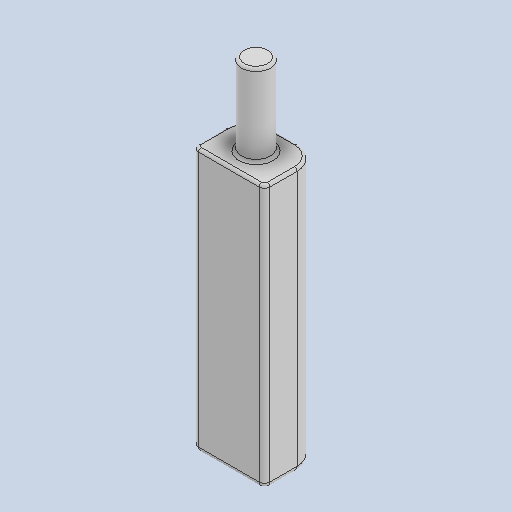
# Autodesk Inventor part: ArmLength
Saved by Autodesk Inventor 2025.2 (Build 292293000, 293)
## iProperties
Created: 2025-02-05
Part Number: ArmLength
Material: Generic
Document SubType Name: Modeling
Designer: andre
Density: 1 g/cm^3
Appearance: Default
Author: andre
Autodesk Inventor part; units mm, degrees
ref_plane "YZ Plane" through (0, 0, 0) normal (1, 0, 0) x (0, 1, 0)
ref_plane "XZ Plane" through (0, 0, 0) normal (0, 1, 0) x (-1, 0, 0)
ref_plane "XY Plane" through (0, 0, 0) normal (0, 0, 1) x (1, 0, 0)
sketch "Sketch1" plane through (0, 0, 0) normal (0, 0, 1) x (1, 0, 0)
  arc A0 (6.6, 0) -> (-2.5948, -6.0685) centre (0, 0) ccw construction
  circle A1 centre (0, 0) radius 6.6
  line L0 (-6.5674, -56.9808) -> (6.5674, -56.9808)
  line L1 (6.5674, -56.9808) -> (6.5674, 56.9808)
  line L2 (6.5674, 56.9808) -> (-6.5674, 56.9808)
  line L3 (-6.5674, 56.9808) -> (-6.5674, -56.9808)
  line L4 (-6.5674, -56.9808) -> (6.5674, 56.9808) construction
  line L5 (6.5674, -56.9808) -> (-6.5674, 56.9808) construction
  line L6 (6.5674, -6.6) -> (-6.5674, -6.6)
  line L7 (-2.8891, -3.8891) -> (2.8891, -3.8891) projected
  arc A2 (2.8891, -3.8891) -> (3.8891, -2.8891) centre (2.8891, -2.8891) ccw projected
  line L8 (3.8891, -2.8891) -> (3.8891, 2.8891) projected
  arc A3 (3.8891, 2.8891) -> (2.8891, 3.8891) centre (2.8891, 2.8891) ccw projected
  line L9 (2.8891, 3.8891) -> (-2.8891, 3.8891) projected
  arc A4 (-2.8891, 3.8891) -> (-3.8891, 2.8891) centre (-2.8891, 2.8891) ccw projected
  line L10 (-3.8891, 2.8891) -> (-3.8891, -2.8891) projected
  arc A5 (-3.8891, -2.8891) -> (-2.8891, -3.8891) centre (-2.8891, -2.8891) ccw projected
  constraints: 14 end point, 2 midpoint, 2 parallel, 2 perpendicular, 2 point on line, 1 centre point, 1 coincident, 1 concentric, 1 horizontal
extrude "Extrusion1" add sketch "Sketch1" along normal blind 10 contours L1 A1 L3 | A1 L3 L2 L1 | L1 L6 A1 | L6 L3 A1 | A5 L10 A4 L9 A3 L8 A2 L7
fillet "Fillet1" radius 4 2 edges at (6.5674, 25.1904, 0) (-6.5674, 25.1904, 0)
fillet "Fillet2" radius 1 2 edges at (6.5674, 25.1904, 10) (-6.5674, 25.1904, 10)
fillet "Fillet3" radius 1 8 edges at (6.2745, -6.6, 9.7071) (6.5674, -6.6, 6.5) (5.3959, -6.6, 1.1716) (0, -6.6, 0) (-5.3959, -6.6, 1.1716) (-6.5674, -6.6, 6.5) (-6.2745, -6.6, 9.7071) (0, -6.6, 10)
sketch "Sketch2" plane through (0, 0, 0) normal (0, 0, -1) x (-1, 0, 0)
  point P0 (0, 0)
sketch "Sketch3" plane through (0, 0, 0) normal (0, 0, -1) x (-1, 0, 0)
  arc A0 (2.8891, -3.8891) -> (3.8891, -2.8891) centre (2.8891, -2.8891) ccw projected
  line L0 (3.8891, -2.8891) -> (3.8891, 2.8891) projected
  arc A1 (3.8891, 2.8891) -> (2.8891, 3.8891) centre (2.8891, 2.8891) ccw projected
  line L1 (2.8891, 3.8891) -> (-2.8891, 3.8891) projected
  arc A2 (-2.8891, 3.8891) -> (-3.8891, 2.8891) centre (-2.8891, 2.8891) ccw projected
  line L2 (-3.8891, 2.8891) -> (-3.8891, -2.8891) projected
  arc A3 (-3.8891, -2.8891) -> (-2.8891, -3.8891) centre (-2.8891, -2.8891) ccw projected
  line L3 (-2.8891, -3.8891) -> (2.8891, -3.8891) projected
  line L4 (2.5948, -6.0685) -> (-6.6, -10) projected
  line L5 (-6.6, -10) -> (-6.6, 0) projected
  arc A4 (2.5948, -6.0685) -> (-6.6, 0) centre (0, 0) ccw projected
extrude "Extrusion2" cut sketch "Sketch3" against normal blind 5 contours L3 A3 L2 A2 L1 A1 L0 A0
fillet "Fillet4" radius 0.5 20 edges at (-3.5962, -3.5962, 5) (0, -3.8891, 5) (3.5962, -3.5962, 5) (3.8891, 0, 5) (3.5962, 3.5962, 5) (0, 3.8891, 5) (-3.5962, 3.5962, 5) (-3.8891, 0, 5) (2.7284, -3.8891, 0.0032) (3.6285, -3.5623, 0.1433) (3.8891, 0, 0.2247) (3.6271, 3.5639, 0.1429) (2.7284, 3.8891, 0.0032) (0, 3.8891, 0) (-2.7284, 3.8891, 0.0032) (-3.6286, 3.5623, 0.1433) (-3.8891, 0, 0.2247) (-3.6283, -3.5626, 0.1432) (-2.7284, -3.8891, 0.0032) (0, -3.8891, 0)
sketch "Sketch4" plane through (-2.5674, 56.9808, 0) normal (0, 1, 0) x (1, 0, 0)
  arc A0 (-4, -9) -> (-3, -10) centre (-3, -9) ccw projected
  line L0 (8.1349, -10) -> (-3, -10) projected
  arc A1 (8.1349, -10) -> (9.1349, -9) centre (8.1349, -9) ccw projected
  line L1 (9.1349, -4) -> (9.1349, -9) projected
  arc A2 (9.1349, -4) -> (5.1349, 0) centre (5.1349, -4) ccw projected
  line L2 (5.1349, 0) -> (0, 0) projected
  arc A3 (0, 0) -> (-4, -4) centre (0, -4) ccw projected
  line L3 (-4, -4) -> (-4, -9) construction
  line L4 (9.1857, -10) -> (-4.0508, -10) construction
  line L5 (-4.0508, -10) -> (-4.0508, 0) construction
  line L6 (-4.0508, 0) -> (9.1857, 0) construction
  line L7 (9.1857, 0) -> (9.1857, -10) construction
  circle A4 centre (2.5674, -5) radius 2.6492
  line L8 (2.5674, 0) -> (2.5674, -10) construction
  line L9 (9.1349, -4) -> (9.1349, -9) construction
  line L10 (9.1349, -5) -> (-4, -5) construction
  line L11 (-4, -9) -> (-4, -4) construction
  line L12 (-4, -4) -> (-4, -9) projected
  dimension "d8" = 5
  constraints: 12 end point, 2 midpoint, 2 parallel, 2 perpendicular, 2 point on line, 1 centre point, 1 coincident, 1 horizontal
  measures "d8" distance between parallel lines of L0 L10
extrude "Extrusion3" cut sketch "Sketch4" against normal blind 15
fillet "Fillet5" radius 0.5 2 edges at (-2.6492, 41.9808, 5) (-2.6492, 56.9808, 5)
fillet "Fillet6" radius 0.5 8 edges at (-6.2745, 41.9808, 9.7071) (-6.5674, 41.9808, 6.5) (-5.3959, 41.9808, 1.1716) (0, 41.9808, 0) (5.3959, 41.9808, 1.1716) (6.5674, 41.9808, 6.5) (6.2745, 41.9808, 9.7071) (0, 41.9808, 10)
body "Solid1"
